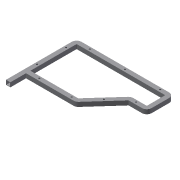
# Autodesk Inventor part: frame
Saved by Autodesk Inventor 2022 (Build 260148000, 148)
## iProperties
Created: 2006-05-17
Part Number: frame
Document SubType Name: Modeling
Designer: dchu
Density: 1 g/cm^3
Material: Generic
Appearance: Default
Author: dchu
Autodesk Inventor part; units mm, degrees
ref_plane "YZ Plane" through (0, 0, 0) normal (1, 0, 0) x (0, 1, 0)
ref_plane "XZ Plane" through (0, 0, 0) normal (0, 1, 0) x (-1, 0, 0)
sketch "Sketch1" plane through (0, 0, 0) normal (0, 0, 1) x (1, 0, 0)
  line L0 (493.3784, 596.83) -> (-506.6216, 596.83)
  line L1 (-536.6216, 566.83) -> (-536.6216, -183.17)
  line L2 (523.3784, 566.83) -> (523.3784, 366.83)
  line L3 (493.3784, 336.83) -> (343.3784, 336.83)
  line L4 (321.0933, 326.9141) -> (53.3048, 29.7789)
  arc A0 (-506.6216, 596.83) -> (-536.6216, 566.83) centre (-506.6216, 566.83) ccw
  arc A1 (523.3784, 566.83) -> (493.3784, 596.83) centre (493.3784, 566.83) ccw
  arc A2 (493.3784, 336.83) -> (523.3784, 366.83) centre (493.3784, 366.83) ccw
  arc A3 (343.3784, 336.83) -> (321.0933, 326.9141) centre (343.3784, 306.83) ccw
  line L5 (31.0196, 19.863) -> (-536.6216, 19.863) construction
  arc A4 (31.0196, 19.863) -> (53.3048, 29.7789) centre (31.0196, 49.863) ccw
  dimension "d0" = 30
  dimension "d1" = 30
  dimension "d3" = 1000
  dimension "d4" = 200
  dimension "d5" = 750
  dimension "d6" = 150
  dimension "d7" = 400
  constraints: 12 end point, 10 point on circle, 10 tangent, 5 centre point, 3 equal radius, 3 perpendicular, 1 horizontal, 1 parallel, 1 point on line
  measures "d0" radius of A0
  measures "d1" radius of A4
  measures "d3" distance of L0.start L0.end
  measures "d4" distance of L2.start L2.end
  measures "d5" distance of L1.start L1.end
  measures "d6" distance of L3.start L3.end
  measures "d7" distance of L4.start L4.end
ref_plane "Work Plane1" through (-536.6216, -183.17, 0) normal (0, 1, 0) x (-1, 0, 0)
sketch "Sketch5" plane through (-536.6216, -183.17, 0) normal (0, 1, 0) x (-1, 0, 0)
  line L0 (24.9153, 23.9725) -> (-25.0847, 23.9725)
  line L1 (-25.0847, 23.9725) -> (-25.0847, -26.0275)
  line L2 (-25.0847, -26.0275) -> (24.9153, -26.0275)
  line L3 (24.9153, -26.0275) -> (24.9153, 23.9725)
  line L4 (19.9153, 18.9725) -> (-20.0847, 18.9725)
  line L5 (-20.0847, 18.9725) -> (-20.0847, -21.0275)
  line L6 (-20.0847, -21.0275) -> (19.9153, -21.0275)
  line L7 (19.9153, -21.0275) -> (19.9153, 18.9725)
  point P0 (0, 0)
  dimension "d8" = 50
  dimension "d9" = 50
  dimension "d10" = 5
  dimension "d12" = 5
  dimension "d13" = 5
  dimension "d14" = 5
  constraints: 16 end point, 4 parallel, 2 horizontal, 2 perpendicular
  measures "d8" distance of L2.end L0.start
  measures "d9" distance of L0.start L0.end
  measures "d10" distance between parallel lines of L3 L7
  measures "d12" distance between parallel lines of L6 L2
  measures "d13" distance between parallel lines of L1 L5
  measures "d14" distance between parallel lines of L0 L4
sweep "Sweep2" add profiles "Sketch5" path "Sketch1"
sketch "Sketch6" plane through (31.0196, -5.0523, -26.0275) normal (-1, 0, 0) x (0, 0, 1)
  line L0 (45, 5) -> (5, 5) projected
  line L1 (5, 5) -> (5, 45) projected
  line L2 (5, 45) -> (45, 45) projected
  line L3 (45, 45) -> (45, 5) projected
  line L4 (0, 0) -> (0, 50) projected
  line L5 (50, 0) -> (0, 0) projected
  line L6 (50, 50) -> (50, 0) projected
  line L7 (0, 50) -> (50, 50) projected
extrude "Extrusion1" add sketch "Sketch6" along normal up to next
sketch "Sketch7" plane through (-561.5369, -183.17, 23.9725) normal (0, 0, 1) x (1, 0, 0)
  line L0 (50, 228.1178) -> (50, 750) projected
  line L1 (54.9153, 754.9153) -> (1054.9153, 754.9153) projected
  line L2 (1054.9153, 545.0847) -> (904.9153, 545.0847) projected
  line L3 (863.9962, 526.8776) -> (596.2078, 229.7424) projected
  line L4 (592.5565, 228.1178) -> (50, 228.1178) projected
  point P0 (175.6092, 779.9153)
  point P1 (575.6092, 779.9153)
  point P2 (975.6092, 781.6554)
  point P3 (963.1788, 520.0847)
  point P4 (545.6092, 203.1178)
  point P5 (175.6092, 203.1178)
  point P6 (25, 660.086)
  point P7 (25, 328.8534)
  point P8 (751.3683, 364.564)
  dimension "d18" = 25
  dimension "d19" = 400
  dimension "d20" = 400
  dimension "d21" = 370
  dimension "d22" = 25
  dimension "d23" = 25
  dimension "d24" = 25
  dimension "d25" = 25
  constraints: 2 horizontal alignment, 2 vertical alignment
  measures "d18" distance from line of L1 point (175.609, 779.915)
  measures "d19" distance of point (575.609, 779.915) point (175.609, 779.915)
  measures "d20" horizontal distance of point (975.609, 781.655) point (575.609, 779.915)
  measures "d21" distance of point (545.609, 203.118) point (175.609, 203.118)
  measures "d22" distance from line of L4 point (545.609, 203.118)
  measures "d23" distance from line of L0 point (25, 660.086)
  measures "d24" distance from line of L2 point (963.179, 520.085)
  measures "d25" distance from line of point (751.368, 364.564) L3
hole "Hole1" at (-385.9276, 596.7452, 23.9725) at (14.0724, 596.7452, 23.9725) at (414.0724, 598.4853, 23.9725) at (401.6419, 336.9147, 23.9725) at (-15.9276, 19.9477, 23.9725) at (-385.9276, 19.9477, 23.9725) at (-536.5369, 476.9159, 23.9725) at (-536.5369, 145.6834, 23.9725) at (189.8315, 181.394, 23.9725) direction (0, 0, -1) diameter 17.294 end through all
body "Solid1"
